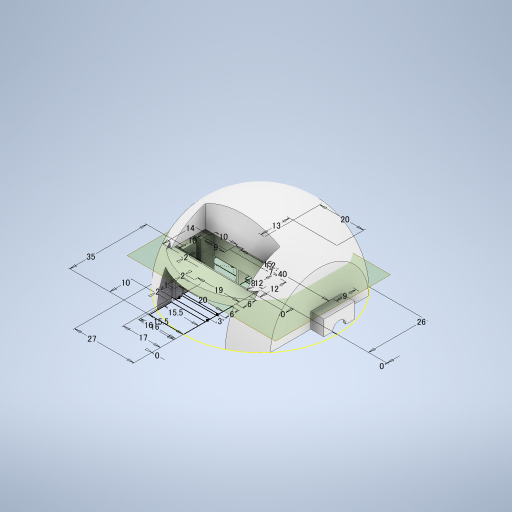
# Autodesk Inventor part: naibu
Saved by Autodesk Inventor 2023 (Build 270158000, 158)
## iProperties
Created: 2022-10-08
Part Number: naibu
Material: ABS プラスチック
Document SubType Name: Modeling
Designer: ellie
Density: 1.06 g/cm^3
Appearance: 積雪
Author: ellie
Autodesk Inventor part; units mm, degrees
ref_plane "YZ Plane" through (0, 0, 0) normal (1, 0, 0) x (0, 1, 0)
ref_plane "XZ Plane" through (0, 0, 0) normal (0, 1, 0) x (-1, 0, 0)
ref_plane "XY Plane" through (0, 0, 0) normal (0, 0, 1) x (1, 0, 0)
sketch "スケッチ1" plane through (0, 0, 0) normal (0, 1, 0) x (-1, 0, 0)
  circle A0 centre (0, 0) radius 35
  line L0 (0, 0) -> (0, -35)
  line L1 (0, 0) -> (0, 35)
  dimension "d0" = 70
  constraints: 4 end point, 2 point on circle, 2 vertical, 1 centre point, 1 coincident
  measures "d0" diameter of A0
revolve "回転1" add sketch "スケッチ1" angle 180 about axis through (0, 0, 0) along (0, 0, 1) picked at (-2.5961, -23.0408) contours L1 L0 A0
sketch "スケッチ5" plane through (0, 0, 0) normal (0, -1, 0) x (1, 0, 0)
  line L0 (-20, -22) -> (20, -22)
  line L1 (20, -22) -> (20, -13)
  line L2 (20, -13) -> (-20, -13)
  line L3 (-20, -13) -> (-20, -22)
  line L4 (-20, -15) -> (-20, -13)
  line L5 (0, 25) -> (-17, 25)
  line L6 (-17, 25) -> (-17, 23)
  line L7 (-17, 23) -> (0, 23)
  line L8 (0, 23) -> (0, 25)
  line L9 (0, 20) -> (-20, 20)
  line L10 (-20, 20) -> (-20, 19)
  line L11 (-20, 19) -> (0, 19)
  line L12 (0, 19) -> (0, 20)
  line L13 (0, 13) -> (-19, 13)
  line L14 (-19, 13) -> (-19, 11)
  line L15 (-19, 11) -> (0, 11)
  line L16 (0, 11) -> (0, 13)
  line L17 (0, 5) -> (-23, 5)
  line L18 (-23, 5) -> (-23, 3)
  line L19 (-23, 3) -> (0, 3)
  line L20 (0, 3) -> (0, 5)
  circle A0 centre (0, 0) radius 35 projected
  circle A1 centre (0, 0) radius 35 projected
  line L21 (0, 35) -> (0, -35)
  line L22 (35, 0) -> (-35, 0)
  line L23 (-32, 2) -> (-23, 2)
  line L24 (-23, 2) -> (-23, -8)
  line L25 (-23, -8) -> (-32, -8)
  line L26 (-32, -8) -> (-32, 2)
  line L27 (-23, -8.0262) -> (-23, 2)
  line L28 (-27, 22.2711) -> (-27, -22.2711)
  line L29 (-15.5, 25) -> (0, 25)
  line L30 (0, 25) -> (0, 35)
  line L31 (0, 35) -> (-15.5, 35)
  line L32 (-15.5, 35) -> (-15.5, 25)
  line L33 (-15.5, 23) -> (0, 23)
  line L34 (0, 23) -> (0, 20)
  line L35 (0, 20) -> (-15.5, 20)
  line L36 (-15.5, 20) -> (-15.5, 23)
  line L37 (-16, 13) -> (0, 13)
  line L38 (0, 13) -> (0, 19)
  line L39 (0, 19) -> (-16, 19)
  line L40 (-16, 19) -> (-16, 13)
  line L41 (-16, 11) -> (0, 11)
  line L42 (0, 11) -> (0, 5)
  line L43 (0, 5) -> (-16, 5)
  line L44 (-16, 5) -> (-16, 11)
  line L45 (-23, -3) -> (-39.6865, -3)
  line L46 (-23, -3) -> (-7.8337, -3)
  line L47 (-8, 3) -> (-23, 3)
  line L48 (-23, 3) -> (-23, -9)
  line L49 (-23, -9) -> (-8, -9)
  line L50 (-8, -9) -> (-8, 3)
  line L51 (-8, 3) -> (-23, -9) construction
  line L52 (-23, 3) -> (-8, -9) construction
  line L53 (-23, 4) -> (-33, 4)
  line L54 (-33, 4) -> (-33, -10)
  line L55 (-33, -10) -> (-23, -10)
  line L56 (-23, -10) -> (-23, 4)
  line L57 (-23, 4) -> (-33, -10) construction
  line L58 (-33, 4) -> (-23, -10) construction
  line L59 (-8, 3) -> (-1, 3)
  line L60 (-1, 3) -> (-1, -9)
  line L61 (-1, -9) -> (-8, -9)
  line L62 (-8, -9) -> (-8, 3)
  line L63 (-8, 3) -> (-1, -9) construction
  line L64 (-1, 3) -> (-8, -9) construction
  line L65 (-23, 2) -> (-27, 2)
  line L66 (-23, -8) -> (-27, -8)
  line L67 (-23, 4) -> (-27, 4)
  line L68 (-23, -10) -> (-27, -10)
  line L69 (23.4307, -26) -> (-23.4307, -26)
  line L70 (-8, 3) -> (-6.8, 3)
  line L71 (-6.8, 3) -> (-6.8, -9)
  line L72 (-6.8, -9) -> (-8, -9)
  line L73 (-8, -9) -> (-8, 3)
  line L74 (-3, 5) -> (0, 5)
  line L75 (0, 20) -> (-4, 20)
  line L76 (-4, 19) -> (0, 19)
  line L77 (0, 19) -> (0, 20)
  line L78 (-6, 5) -> (-1, 5)
  line L79 (-1, 3) -> (-6, 3)
  point P0 (0, -22)
  point P1 (0, -13)
  point P2 (0, 24)
  point P3 (0, 19.5)
  point P4 (0, 12)
  point P5 (0, 4)
  point P6 (-20, -17.5)
  point P7 (-27, -0.5262)
  point P8 (-27, -8)
  point P9 (-15.5, 21.5)
  point P10 (-15.5, 31.3807)
  point P11 (0, 25)
  point P12 (0, 23)
  point P13 (0, 11)
  point P14 (0, 13)
  point P15 (-27, 0)
  point P16 (-32, 0)
  point P17 (-23, 0)
  point P18 (-15.5, -3)
  point P19 (-28, -3)
  point P20 (-4.5, -3)
  point P21 (-8, -9)
  point P22 (-8, 3)
  point P23 (-27, 0.5)
  point P24 (-28, 0.4738)
  point P25 (-28, -11.5262)
  point P26 (-27, -11.5)
  point P27 (-23, 2)
  point P28 (-23, 2)
  point P29 (-8, 0)
  point P30 (-1, 0)
  point P31 (0, 19)
  point P32 (0, 20)
  point P33 (-27, -10)
  point P34 (-27, 4)
  dimension "d12" = 40
  dimension "d13" = 9
  dimension "d23" = 17
  dimension "d24" = 2
  dimension "d27" = 20
  dimension "d28" = 1
  dimension "d30" = 19
  dimension "d31" = 2
  dimension "d33" = 2
  dimension "d88" = 0
  dimension "d89" = 0
  dimension "d90" = 13
  dimension "d92" = 20
  dimension "d93" = 10
  dimension "d97" = 9
  dimension "d98" = 10
  dimension "d113" = 27
  dimension "d122" = 15.5
  dimension "d123" = 35
  dimension "d124" = 3
  dimension "d125" = 15.5
  dimension "d126" = 6
  dimension "d127" = 6
  dimension "d128" = 16
  dimension "d129" = 16
  dimension "d147" = 12
  dimension "d149" = 8
  dimension "d151" = 15
  dimension "d161" = 14
  dimension "d162" = 10
  dimension "d164" = 12
  dimension "d165" = 7
  dimension "d170" = 26
  dimension "d175" = 1.2
  dimension "d207" = 0
  constraints: 158 end point, 31 parallel, 20 horizontal, 17 perpendicular, 16 point on line, 15 midpoint, 10 collinear, 1 vertical, 20 other
  measures "d12" distance of L2.end L1.end
  measures "d13" distance of L1.end L0.end
  measures "d23" distance of L7.end L6.end
  measures "d24" distance of L6.end L5.end
  measures "d27" distance of L11.end L10.end
  measures "d28" distance of L10.end L9.end
  measures "d30" distance of L15.end L14.end
  measures "d31" distance of L14.end L13.end
  measures "d33" distance of L18.end L17.end
  measures "d89" distance from line of point (0, 0) L22
  measures "d90" distance from line of L0 point (0, -35)
  measures "d92" distance of the line from the sketch origin of L3
  measures "d93" distance from line of L5 point (0, 35)
  measures "d97" distance of L24.end L25.end
  measures "d98" distance of L23.end L24.end
  measures "d113" distance of the line from the sketch origin of L28
  measures "d122" distance of the line from the sketch origin of L32
  measures "d123" distance between parallel lines of L31 L22
  measures "d124" distance of L33.end L34.end
  measures "d126" distance of L38.end L37.end
  measures "d127" distance of L41.end L42.end
  measures "d128" distance of the line from the sketch origin of L44
  measures "d129" distance of the line from the sketch origin of L40
  measures "d147" distance of L48.end L47.end
  measures "d149" distance of the line from the sketch origin of L50
  measures "d151" distance between parallel lines of L50 L24
  measures "d161" distance between parallel lines of L55 L53
  measures "d162" distance between parallel lines of L48 L54
  measures "d164" distance between parallel lines of L61 L59
  measures "d165" distance between parallel lines of L50 L60
  measures "d170" distance between parallel lines of L69 L22
  measures "d175" distance of L71.end L72.end
  measures "d207" distance between parallel lines of L47 L19
extrude "GNSボード" cut sketch "スケッチ5" against normal blind 16 contours L8 L7 L6 L5
extrude "GNSボード止めるよう" cut sketch "スケッチ5" against normal blind 15 contours L21 L5 L32 A0 | L21 L9 L36 L7
extrude "アルミ板１" cut sketch "スケッチ5" against normal blind 17.5 contours L11 L10 L9 L12
extrude "メイン基板" cut sketch "スケッチ5" against normal blind 17.5 contours L15 L14 L13 L16
extrude "メイン止めるよう" cut sketch "スケッチ5" against normal blind 17.5 contours L17 L44 L15 L21 | L13 L40 L11 L21
extrude "アルミ板２" cut sketch "スケッチ5" against normal blind 19.5 contours L19 L18 L17 L20
extrude "電池ボックス入れ" cut sketch "スケッチ5" against normal blind 15 contours L3 L2 L21 L0 | L21 L2 L1 L0
extrude "side ut" cut sketch "スケッチ5" against normal blind 100 contours A0 L45 L54 L55 L28 | A0 L22 L54 L45 | L55 L54 L45 L26 L25 L28 | A0 L28 L53 L54 L22 | L54 L22 L26 L45 | L25 L26 L45 L28 | L54 L53 L28 L23 L26 L22 | L26 L22 L28 L45 | L22 L26 L23 L28
extrude "motor case" add sketch "スケッチ5" against normal blind 7 contours L55 L54 L45 L26 L25 L28 | L28 L25 L27 L48 L56 L55 | L50 L46 L24 L22 | L22 L24 L48 L19 L50 | L54 L22 L26 L45 | L28 L45 L24 L25 | L25 L26 L45 L28 | L24 L45 L28 L22 | L22 L28 L23 L24 | L50 L49 L48 L27 L24 L46 | L54 L53 L28 L23 L26 L22 | L26 L22 L28 L45 | L53 L18 L48 L23 L28 | L22 L26 L23 L28
extrude "bottom cut" cut sketch "スケッチ5" against normal blind 90 contours L69 A0 L21 | L21 A0 L69
extrude "motor" cut sketch "スケッチ5" against normal blind 6 contours L60 L61 L71 L22 | L22 L71 L19 L60 | L71 L61 L50 L22 | L22 L50 L19 L71 | L50 L46 L24 L22 | L22 L24 L48 L19 L50 | L28 L45 L24 L25 | L25 L26 L45 L28 | L24 L45 L28 L22 | L22 L28 L23 L24 | L50 L49 L48 L27 L24 L46 | L26 L22 L28 L45 | L22 L26 L23 L28
extrude "motor block" add sketch "スケッチ5" against normal blind 10 contours L71 L61 L50 L22 | L22 L50 L19 L71
sketch "スケッチ27" plane through (-33, 0, -10) normal (-1, 0, 0) x (0, 0, 1)
  line L0 (14, 0) -> (0, 0) projected
  circle A0 centre (7, 0) radius 3
  point P0 (10, 0)
  dimension "d198" = 6
  constraints: 1 centre point, 1 midpoint
  measures "d198" diameter of A0
extrude "押し出し36" cut sketch "スケッチ27" against normal blind 27
mirror "ミラー13" about plane through (0, 0, 0) normal (1, 0, 0) of "メイン止めるよう", "メイン基板", "アルミ板１", "GNSボード止めるよう", "GNSボード", "アルミ板２", "motor", "motor case", "押し出し36", "電池ボックス入れ", "side ut", "motor block"
ref_plane "作業平面5" through (-17, 17.5, 23) normal (0, -1, 0) x (1, 0, 0)
sketch "スケッチ29" plane through (-17, 17.5, 23) normal (0, -1, 0) x (1, 0, 0)
  line L0 (32.5, 2) -> (1.5, 2) projected
  line L1 (1.5, 0) -> (32.5, 0) projected
  line L2 (32.5, -3) -> (1.5, -3) projected
  line L3 (1, -4) -> (33, -4) projected
  line L4 (-2, -10) -> (1, -10) projected
  line L5 (33, -10) -> (33, -4) projected
  line L6 (1, -4) -> (-3, -4) projected
  line L7 (1, -10) -> (1, -4) projected
  line L8 (1, -12) -> (33, -12) projected
  line L9 (33, -18) -> (1, -18) projected
  line L10 (33, -18) -> (33, -12) projected
  line L11 (1, -12) -> (-2, -12) projected
  line L12 (1, -18) -> (1, -12) projected
  line L13 (18, -20) -> (40, -20) projected
  line L14 (-6, -20) -> (17, -20) projected
  line L15 (17, -18) -> (-6, -18) projected
  line L16 (-16, -23) -> (-15, -23) projected
  line L17 (-15, -23) -> (-15, -21) projected
  line L18 (-15, -21) -> (-6, -21) projected
  line L19 (-6, -21) -> (-6, -18) projected
  line L20 (-6, -18) -> (1, -18) projected
  line L21 (1, -18) -> (1, -12) projected
  line L22 (1, -12) -> (-2, -12) projected
  line L23 (-2, -12) -> (-2, -10) projected
  line L24 (-2, -10) -> (1, -10) projected
  line L25 (1, -10) -> (1, -4) projected
  line L26 (1, -4) -> (-3, -4) projected
  line L27 (-3, -4) -> (-3, -3) projected
  line L28 (-3, -3) -> (1.5, -3) projected
  line L29 (1.5, -3) -> (1.5, 0) projected
  line L30 (1.5, 0) -> (0, 0) projected
  line L31 (0, 0) -> (0, 2) projected
  line L32 (0, 2) -> (1.5, 2) projected
  line L33 (1.5, 2) -> (1.5, 8.3807) projected
  arc A0 (1.5, 8.3807) -> (-10, -0.7289) centre (17, -23) ccw projected
  line L34 (-10, -0.7289) -> (-10, -19) projected
  line L35 (-10, -19) -> (-16, -19) projected
  line L36 (-16, -19) -> (-16, -23) projected
  line L37 (49, -23) -> (50, -23) projected
  line L38 (50, -19) -> (50, -23) projected
  line L39 (44, -19) -> (50, -19) projected
  line L40 (44, -19) -> (44, -0.7289) projected
  arc A1 (44, -0.7289) -> (32.5, 8.3807) centre (17, -23) ccw projected
  line L41 (32.5, 8.3807) -> (32.5, 2) projected
  line L42 (32.5, 2) -> (34, 2) projected
  line L43 (34, 2) -> (34, 0) projected
  line L44 (34, 0) -> (32.5, 0) projected
  line L45 (32.5, 0) -> (32.5, -3) projected
  line L46 (32.5, -3) -> (37, -3) projected
  line L47 (37, -3) -> (37, -4) projected
  line L48 (37, -4) -> (33, -4) projected
  line L49 (33, -4) -> (33, -10) projected
  line L50 (33, -10) -> (36, -10) projected
  line L51 (36, -10) -> (36, -12) projected
  line L52 (36, -12) -> (33, -12) projected
  line L53 (33, -12) -> (33, -18) projected
  line L54 (33, -18) -> (40, -18) projected
  line L55 (40, -18) -> (40, -21) projected
  line L56 (40, -21) -> (49, -21) projected
  line L57 (49, -21) -> (49, -23) projected
  line L58 (40, -18) -> (-6, -18) projected
  circle A2 centre (17, -23) radius 35 projected
  line L59 (17, -23) -> (17, 12)
  circle A3 centre (17, -23) radius 35
  line L60 (0, 12) -> (34, 12)
  line L61 (34, 12) -> (34, -15)
  line L62 (34, -15) -> (0, -15)
  line L63 (0, -15) -> (0, 12)
  line L64 (37, -3) -> (-3, -3) projected
  line L65 (-3, -4) -> (-3, -3) projected
  line L66 (1, -4) -> (-3, -4) projected
  line L67 (1, -10) -> (1, -4) projected
  line L68 (-2, -10) -> (1, -10) projected
  line L69 (-2, -12) -> (-2, -10) projected
  line L70 (33, -12) -> (36, -12) projected
  line L71 (36, -12) -> (36, -10) projected
  line L72 (36, -10) -> (33, -10) projected
  line L73 (33, -10) -> (33, -4) projected
  line L74 (33, -4) -> (37, -4) projected
  line L75 (37, -4) -> (37, -3) projected
  line L76 (37, -3) -> (-3, -3) projected
  line L77 (-3, -4) -> (-3, -3) projected
  line L78 (-2, -12) -> (-2, -10) projected
  line L79 (1, -12) -> (-2, -12) projected
  line L80 (1, -18) -> (1, -12) projected
  line L81 (33, -18) -> (1, -18) projected
  line L82 (33, -18) -> (33, -12) projected
  line L83 (33, -12) -> (36, -12) projected
  line L84 (36, -12) -> (36, -10) projected
  line L85 (36, -10) -> (33, -10) projected
  line L86 (33, -4) -> (37, -4) projected
  line L87 (37, -4) -> (37, -3) projected
  point P0 (37, -3)
  point P1 (34, -10)
  point P2 (34, -12)
  point P3 (34, -4)
  point P4 (34, -3)
  point P5 (34, 0)
  point P6 (0, -3)
  point P7 (0, -4)
  point P8 (0, -10)
  point P9 (0, -12)
  point P10 (1, -15)
  point P11 (33, -15)
  point P12 (34, 0)
  dimension "d217" = 3
  dimension "d218" = 6
  dimension "d219" = 6
  constraints: 10 end point, 2 parallel, 1 centre point, 1 coincident, 1 concentric, 1 horizontal, 1 perpendicular, 1 point on circle, 1 tangent, 1 vertical
  measures "d217" distance between parallel lines of L62 L9
  measures "d218" distance between parallel lines of L63 L19
  measures "d219" distance between parallel lines of L61 L55
extrude "押し出し38" cut sketch "スケッチ29" against normal blind 100 contours L42 L43 L44 L1 L59 L0 | L0 L59 A2 L41 | L41 A1 L61 L42 | L59 L1 L30 L31 L32 L0 | L0 L33 A2 L59 | A2 L60 L61 A1 | L32 L63 A0 L33 | L59 L2 L29 L1 | L1 L45 L2 L59 | A2 A0 L63 L60 | L61 L46 L45 L44 | L29 L28 L63 L30 | L59 L3 L6 L63 L28 L2 | L2 L46 L61 L48 L3 L59 | L59 L8 L11 L63 L4 L7 L3 | L3 L5 L50 L61 L52 L8 L59 | L61 L50 L5 L48 | L7 L4 L63 L6 | L59 L62 L12 L8 | L8 L10 L62 L59 | L12 L62 L63 L11 | L52 L61 L62 L10
sketch "スケッチ33" plane through (-17, 17.5, 8) normal (0, 0, 1) x (1, 0, 0)
  line L0 (-3, -17.5) -> (-3, 0) projected
  line L1 (-3, 0) -> (40, 0)
  line L2 (40, 0) -> (40, 2)
  line L3 (40, 2) -> (-3, 2)
  line L4 (-3, 2) -> (-3, 0)
  point P0 (17, -17.5)
  dimension "d220" = 2
  dimension "d225" = 43
  constraints: 8 end point, 2 parallel, 1 horizontal, 1 perpendicular
  measures "d220" distance of L2.end L1.end
  measures "d225" distance between parallel lines of L2 L4
extrude "押し出し40" cut sketch "スケッチ33" against normal blind 3
sketch "スケッチ35" plane through (-17, 17.5, 19) normal (1, 0, 0) x (0, 0, -1)
  arc A0 (11, 12.0296) -> (-6.0948, 0) centre (19, -17.5) ccw projected
  line L0 (-6.0948, 0) -> (-1, 0) projected
  line L1 (0, 0) -> (-1, 0) projected
  line L2 (0, 0) -> (6, 0) projected
  line L3 (8, 0) -> (6, 0) projected
  line L4 (8, 0) -> (11, 0) projected
  line L5 (11, 0) -> (11, 2) projected
  line L6 (11, 2) -> (11, 12.0296) projected
  line L7 (11, 2) -> (-7.1849, 2)
  line L8 (-7.1849, 2) -> (-7.1849, 0)
  line L9 (-7.1849, 0) -> (11, 0)
  line L10 (11, 0) -> (11, 2)
  point P0 (-4.5744, 2)
  constraints: 8 end point, 2 parallel, 1 horizontal, 1 perpendicular
extrude "押し出し42" cut sketch "スケッチ35" against normal blind 3 contours L7 L5 L4 L3 L2 L1 L0 A0
sketch "スケッチ36" plane through (17, 17.5, 13) normal (-1, 0, 0) x (0, 0, 1)
  line L0 (-5, 0) -> (-2, 0) projected
  line L1 (-5, 0) -> (15.7903, 0)
  line L2 (15.7903, 0) -> (15.7903, 2.3626)
  line L3 (15.7903, 2.3626) -> (-5, 2.3626)
  line L4 (-5, 2.3626) -> (-5, 0)
  point P0 (-13, -17.5)
  constraints: 8 end point, 2 parallel, 1 horizontal, 1 perpendicular
extrude "押し出し43" cut sketch "スケッチ36" against normal blind 3
